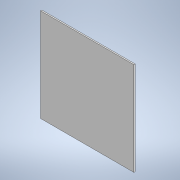
# Autodesk Inventor part: CaseBottom
Saved by Autodesk Inventor 2020.1 (Build 241239000, 239)
## iProperties
Created: 2019-09-03
Part Number: CaseBottom
Material: Generic
Document SubType Name: Modeling
Designer: matteo.spadetto-1
Density: 1 g/cm^3
Appearance: Default
Author: matteo.spadetto-1
Autodesk Inventor part; units mm, degrees
ref_plane "YZ Plane" through (0, 0, 0) normal (1, 0, 0) x (0, 1, 0)
ref_plane "XZ Plane" through (0, 0, 0) normal (0, 1, 0) x (-1, 0, 0)
ref_plane "XY Plane" through (0, 0, 0) normal (0, 0, 1) x (1, 0, 0)
sketch "Sketch1" plane through (0, 0, 0) normal (0, 0, 1) x (1, 0, 0)
  line L0 (0, 0) -> (65, 0)
  line L1 (65, 0) -> (65, 65)
  line L2 (65, 65) -> (0, 65)
  line L3 (0, 65) -> (0, 0)
  dimension "d0" = 65
  dimension "d1" = 65
  constraints: 8 end point, 2 parallel, 1 horizontal, 1 perpendicular
  measures "d0" distance of L2.end L1.end
  measures "d1" distance of L1.end L0.end
extrude "Extrusion1" add sketch "Sketch1" along normal blind 2.3
sketch "Sketch2" plane through (0, 0, 2.3) normal (0, 0, 1) x (1, 0, 0)
  line L0 (-4, 69) -> (69, 69)
  line L1 (69, 69) -> (69, -4)
  line L2 (69, -4) -> (-4, -4)
  line L3 (-4, -4) -> (-4, 69)
  point P0 (0, 0)
  point P1 (0, 65)
  point P2 (65, 0)
  constraints: 8 end point, 2 parallel, 1 perpendicular
extrude "Extrusion2" add sketch "Sketch2" along normal blind 1
sketch "Sketch3" plane through (0, 0, 0) normal (0, 0, -1) x (-1, 0, 0)
  line L0 (0, 0) -> (-65, 0) projected
  line L1 (0, 65) -> (0, 0) projected
  line L2 (-65, 0) -> (-65, 65) projected
  line L3 (-52, 65) -> (-52, 26)
  line L4 (-52, 26) -> (0, 26)
  line L5 (-51, 27) -> (-51, 65)
  line L6 (-51, 65) -> (-52, 65)
  line L7 (0, 65) -> (-1, 65)
  line L8 (-51, 27) -> (0, 27)
  point P0 (0, 26)
  constraints: 12 end point, 3 perpendicular, 1 horizontal, 1 parallel, 1 point on line
extrude "Extrusion5" add sketch "Sketch3" along normal blind 1
sketch "Sketch6" plane through (0, 0, 0) normal (0, 0, -1) x (-1, 0, 0)
  line L0 (-65, 65) -> (-52, 65) projected
  line L1 (-65, 55.5) -> (-52, 55.5)
  line L2 (-52, 26) -> (-52, 65) projected
  line L3 (-52, 55.5) -> (-52, 9.5)
  line L4 (-52, 9.5) -> (-65, 9.5)
  line L5 (-65, 9.5) -> (-65, 55.5)
  line L6 (-65, 0) -> (-65, 65) projected
  point P0 (0, 0)
  dimension "d23" = 46
  constraints: 8 end point, 2 collinear, 1 point on line
  measures "d23" distance of L1.end L3.end
extrude "Extrusion6" cut sketch "Sketch6" against normal blind 3 contours L1 L2 L3 L4 L5
sketch "Sketch7" plane through (0, 0, 0) normal (0, 0, -1) x (-1, 0, 0)
  line L0 (-65, 9.5) -> (-65, 55.5) projected
  line L1 (-52, 55.5) -> (-52, 65) projected
  line L2 (-52, 55.5) -> (-65, 55.5)
  line L3 (-65, 55.5) -> (-65, 58.5)
  line L4 (-65, 58.5) -> (-52, 58.5)
  line L5 (-52, 58.5) -> (-52, 55.5)
  point P0 (0, 0)
  constraints: 8 end point, 2 parallel, 1 horizontal, 1 perpendicular
extrude "Extrusion7" cut sketch "Sketch7" against normal blind 3
body "Solid1"
